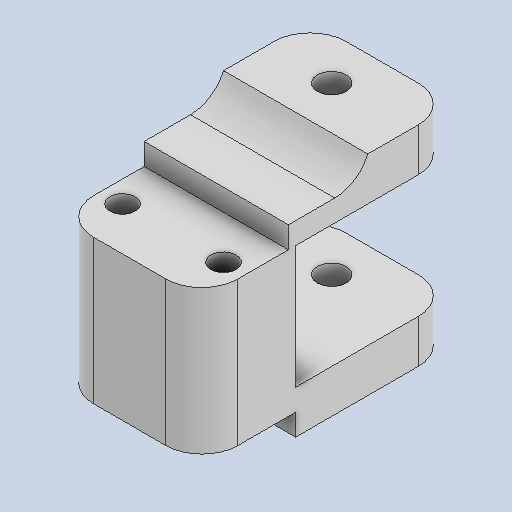
# Autodesk Inventor part: support_avant
Saved by Autodesk Inventor 2024 (Build 280153000, 153)
## iProperties
Created: 2021-11-10
Part Number: support_avant
Material: Générique
Document SubType Name: Modeling
Designer: ropertth
Density: 1 g/cm^3
Appearance: Par défaut
Mass: 10.4128 g
Surface Area: 46.2652 cm^2
Volume: 10.4128 cm^3
Author: ropertth
## iProperties of the stored document support_avant_3DPrint.ipt
Created: 2022-11-21
Part Number: support_avant_3DPrint
Material: Generic
Document SubType Name: Modeling
Designer: Thomas
Density: 1 g/cm^3
Appearance: Default
Author: Thomas
Autodesk Inventor part; units mm, degrees
ref_plane "YZ Plane" through (0, 0, 0) normal (1, 0, 0) x (0, 1, 0)
ref_plane "XZ Plane" through (0, 0, 0) normal (0, 1, 0) x (-1, 0, 0)
ref_plane "XY Plane" through (0, 0, 0) normal (0, 0, 1) x (1, 0, 0)
sketch "Esquisse1" plane through (0, 0, 0) normal (1, 0, 0) x (0, 1, 0)
  line L0 (3, 0) -> (23, 0)
  line L1 (23, 0) -> (23, -12)
  line L2 (23, -12) -> (26, -12)
  line L3 (26, -12) -> (26, -23)
  line L4 (29, -35) -> (23, -35)
  line L5 (23, -35) -> (23, -18)
  line L6 (23, -18) -> (6, -18)
  line L7 (6, -18) -> (6, -35)
  line L8 (6, -35) -> (0, -35)
  line L9 (26, -23) -> (29, -23)
  line L10 (29, -23) -> (29, -35)
  line L11 (3, 0) -> (3, -13)
  line L12 (3, -13) -> (0, -13)
  line L13 (0, -13) -> (0, -35)
  point P0 (0, 0)
  dimension "d0" = 35
  dimension "d2" = 17
  dimension "d4" = 17
  dimension "d6" = 3
  dimension "d7" = 12
  dimension "d8" = 12
  dimension "d10" = 3
  dimension "d34" = 13
  dimension "d35" = 3
  dimension "d36" = 29
  dimension "d37" = 6
  dimension "d38" = 0
  dimension "d44" = 0
  constraints: 28 end point, 10 perpendicular, 2 horizontal, 2 point on line, 1 vertical
  measures "d0" distance between parallel lines of L4 L0
  measures "d2" distance between parallel lines of L5 L7
  measures "d4" distance of L4.end L5.end
  measures "d6" distance between parallel lines of L3 L1
  measures "d7" distance of L0.end L1.end
  measures "d8" distance of L9.end L4.start
  measures "d10" distance of L3.end L9.end
  measures "d34" distance of L0.start L11.end
  measures "d35" distance of L11.end L12.end
  measures "d36" distance between parallel lines of L13 L10
  measures "d37" distance of L4.start L4.end
  measures "d38" distance from line of L13 point (0, 0)
  measures "d44" distance from line of point (0, 0) L0
extrude "Extrusion1" add sketch "Esquisse1" along normal blind 20
sketch "Esquisse2" plane through (0, 29, -23) normal (0, 1, 0) x (1, 0, 0)
  line L0 (0, 12) -> (20, 12) projected
  line L1 (20, 12) -> (20, 0) projected
  point P0 (0, -23)
  point P1 (9, 6)
  dimension "d20" = 6
  dimension "d21" = 11
  measures "d20" distance from line of L0 point (9, 6)
  measures "d21" distance from line of L1 point (9, 6)
hole "Perçage1" at (9, 29, -29) direction (0, -1, 0) diameter 4 end through all
sketch "Esquisse3" plane through (0, 23, 0) normal (0, 1, 0) x (1, 0, 0)
  line L0 (0, 0) -> (20, 0) projected
  line L1 (0, 12) -> (0, 0) projected
  point P0 (3, 6)
  dimension "d29" = 6
  dimension "d30" = 3
  measures "d29" distance from line of L0 point (3, 6)
  measures "d30" distance from line of L1 point (3, 6)
hole "Perçage2" at (3, 23, -6) direction (0, -1, 0) diameter 3.5 end through all
pattern_linear "Réseau rectangulaire1" count 2 spacing 14 along (1, 0, 0) of "Perçage2"
chamfer "Chanfrein1" distance 5 angle 45 2 edges at (0, 14.5, -18) (20, 14.5, -18)
fillet "Congé1" radius 5 6 edges at (0, 26, -35) (20, 26, -35) (0, 3, -35) (20, 3, -35) (20, 13, 0) (0, 13, 0)
fillet "Congé2" radius 5 1 edges at (10, 26, -23)
